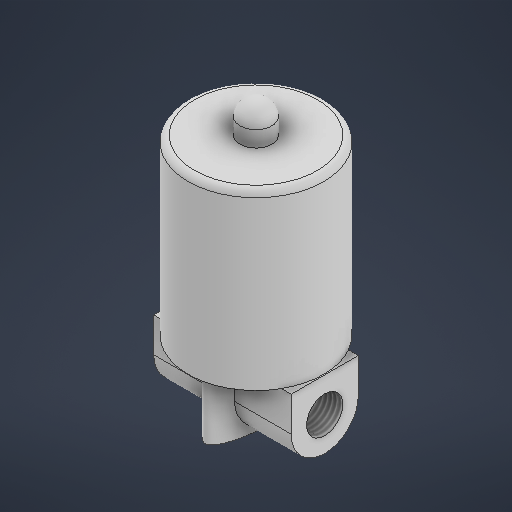
# Autodesk Inventor part: ElectronicValve
Saved by Autodesk Inventor 2026.2 (Build 302298000, 298)
## iProperties
Created: 2026-01-18
Part Number: ElectronicValve
Material: Generic
Document SubType Name: Modeling
Designer: User
Density: 1 g/cm^3
Appearance: Default
Author: User
Autodesk Inventor part; units mm, degrees
ref_plane "YZ Plane" through (0, 0, 0) normal (1, 0, 0) x (0, 1, 0)
ref_plane "XZ Plane" through (0, 0, 0) normal (0, 1, 0) x (-1, 0, 0)
ref_plane "XY Plane" through (0, 0, 0) normal (0, 0, 1) x (1, 0, 0)
sketch "Sketch1" plane through (0, 0, 0) normal (1, 0, 0) x (0, 1, 0)
  line L0 (0, 0) -> (54.2, 0)
  line L1 (54.2, 0) -> (54.2, 19.2)
  line L2 (52.2, 21.2) -> (0, 21.2)
  line L3 (0, 21.2) -> (0, 0)
  arc A0 (54.2, 19.2) -> (52.2, 21.2) centre (52.2, 19.2) ccw
  point P0 (54.2, 21.2)
  dimension "d0" = 21.2
  dimension "d1" = 54.2
  dimension "d2" = 2
  constraints: 8 end point, 2 parallel, 2 point on circle, 2 point on line, 2 tangent, 1 centre point, 1 horizontal, 1 perpendicular
  measures "d0" distance of L0.end point (54.2, 21.2)
  measures "d1" distance of point (54.2, 21.2) L2.end
  measures "d2" radius of A0
revolve "Revolution1" add sketch "Sketch1" angle 360 about axis through (0, 0, 0) along (0, 1, 0)
sketch "Sketch2" plane through (0, 0, 0) normal (1, 0, 0) x (0, 1, 0)
  line L0 (54.2, -19.2) -> (54.2, 19.2) projected
  line L1 (54.2, 0) -> (64.2, 0)
  line L2 (64.2, 0) -> (64.2, 0)
  line L3 (59.2, 5) -> (54.2, 5)
  line L4 (54.2, 5) -> (54.2, 0)
  arc A0 (64.2, 0) -> (59.2, 5) centre (59.2, 0) ccw
  point P0 (0, 0)
  point P1 (64.2, 5)
  dimension "d4" = 10
  dimension "d5" = 5
  dimension "d6" = 5
  constraints: 8 end point, 2 parallel, 2 point on circle, 2 point on line, 2 tangent, 1 centre point, 1 horizontal, 1 midpoint, 1 perpendicular
  measures "d4" distance of point (64.2, 5) L3.end
  measures "d5" distance of L1.end point (64.2, 5)
  measures "d6" radius of A0
revolve "Revolution2" add sketch "Sketch2" angle 360 about axis through (0, 54.2, 0) along (0, 1, 0)
sketch "Sketch3" plane through (0, 0, 0) normal (1, 0, 0) x (0, 1, 0)
  line L0 (0, 10.5) -> (-21.3, 10.5)
  line L1 (-21.3, 10.5) -> (-21.3, -10.5)
  line L2 (-21.3, -10.5) -> (0, -10.5)
  line L3 (0, -10.5) -> (0, 10.5)
  line L4 (0, 21.2) -> (52.2, 21.2) projected
  line L5 (0, -21.2) -> (52.2, -21.2) projected
  point P0 (0, 0)
  dimension "d8" = 21.3
  dimension "d9" = 21
  dimension "d10" = 10.7
  constraints: 8 end point, 2 parallel, 1 horizontal, 1 midpoint, 1 perpendicular
  measures "d8" distance of L0.start L0.end
  measures "d9" distance of L0.end L1.end
  measures "d10" distance between parallel lines of L4 L0
extrude "Extrusion1" add sketch "Sketch3" along normal mid plane 43
fillet "Fillet1" radius 10.5 2 edges at (0, -21.3, 10.5) (0, -21.3, -10.5)
sketch "Sketch4" plane through (21.5, 0, 0) normal (1, 0, 0) x (0, 0, -1)
  arc A0 (-10.5, -10.8) -> (10.5, -10.8) centre (0, -10.8) ccw projected
  point P0 (0, 0)
  constraints: 1 coincident
hole "Hole1" at (21.5, -10.8, 0) direction (-1, 0, 0) diameter 10.7188 depth 17.076 taper from width 11.3583 to width 10.7323 over 10.0203 thread size "1/4" designation "1/4 - 18 NPT" standard "NPT"
sketch "Sketch5" plane through (-21.5, 0, 0) normal (-1, 0, 0) x (0, 0, 1)
  arc A0 (-10.5, -10.8) -> (10.5, -10.8) centre (0, -10.8) ccw projected
  point P0 (0, 0)
  constraints: 1 coincident
hole "Hole2" at (-21.5, -10.8, 0) direction (1, 0, 0) diameter 10.7188 depth 17.076 taper from width 11.3583 to width 10.7323 over 10.02 thread size "1/4" designation "1/4 - 18 NPT" standard "NPT"
ref_plane "Work Plane1" through (0, -21.3, 0) normal (0, -1, 0) x (1, 0, 0)
sketch "Sketch6" plane through (0, -21.3, 0) normal (0, -1, 0) x (1, 0, 0)
  circle A0 centre (0, 0) radius 5 projected
  ellipse E0 centre (0, 0) end of major axis (0, 16) minor radius 5
  line L0 (21.5, 10.5) -> (-21.5, 10.5) projected
  dimension "d33" = 16
  dimension "d34" = 5
  constraints: 1 coincident, 1 horizontal, 2 other
extrude "Extrusion2" add sketch "Sketch6" against normal blind 21.3
sketch "Sketch7" plane through (0, -21.3, 0) normal (0, -1, 0) x (1, 0, 0)
  circle A0 centre (0, -10.5) radius 2.5
  circle A1 centre (0, 10.5) radius 2.5
  point P0 (0, 0)
  dimension "d37" = 21
  dimension "d38" = 0
  dimension "d39" = 5
  dimension "d40" = 5
  dimension "d41" = 0
  dimension "d42" = 10.5
  constraints: 2 centre point
  measures "d37" distance of A1.centre A0.centre
  measures "d38" horizontal distance of A1.centre A0.centre
  measures "d39" diameter of A0
  measures "d40" diameter of A1
  measures "d41" horizontal distance of point (0, 0) A1.centre
  measures "d42" distance of point (0, 0) A0.centre
hole "Hole3" at (0, -21.3, -10.5) at (0, -21.3, 10.5) direction (0, 1, 0) diameter 4.134 depth 14.2 thread size "M5x0.8" class "6H" standard "ANSI Metric M Profile"
body "Solid1"
